Autodesk Inventor part; units mm, degrees
(part 3 of 3)
  dimension "d58" = 1
  dimension "d59" = 0.5
  dimension "d60" = 6
  dimension "d61" = 7
  dimension "d62" = 1
  dimension "d63" = 0.5
  dimension "d64" = 6
  dimension "d65" = 7
  dimension "d66" = 1
  dimension "d67" = 0.5
  dimension "d68" = 6
  dimension "d69" = 7
  dimension "d70" = 0.5
  dimension "d71" = 1
  dimension "d72" = 7
  dimension "d73" = 6
  dimension "d74" = 1
  dimension "d75" = 0.5
  dimension "d76" = 6
  dimension "d77" = 7
  dimension "d78" = 1
  dimension "d79" = 0.5
  dimension "d80" = 6
  dimension "d81" = 7
  dimension "d82" = 1
  dimension "d83" = 0.5
  constraints: 60 other
  measures "d20" distance of L2.end L0.start
  measures "d21" distance of L1.end L2.end
  measures "d22" distance between parallel lines of L4 L0
  measures "d23" distance between parallel lines of L5 L3
  measures "d24" distance of L8.end L6.start
  measures "d25" distance of L7.end L8.end
  measures "d26" distance between parallel lines of L10 L6
  measures "d27" distance between parallel lines of L11 L9
  measures "d28" distance of L14.end L12.start
  measures "d29" distance of L12.start L12.end
  measures "d30" distance between parallel lines of L16 L12
  measures "d31" distance between parallel lines of L17 L15
  measures "d32" distance of L20.end L18.start
  measures "d33" distance of L19.end L20.end
  measures "d34" distance between parallel lines of L22 L18
  measures "d35" distance between parallel lines of L23 L21
  measures "d36" distance of L25.end L26.end
  measures "d37" distance of L26.end L24.start
  measures "d38" distance between parallel lines of L28 L24
  measures "d39" distance between parallel lines of L29 L27
  measures "d40" distance of L30.start L30.end
  measures "d41" distance of L30.end L31.end
  measures "d42" distance between parallel lines of L34 L30
  measures "d43" distance between parallel lines of L35 L33
  measures "d44" distance of L37.end L38.end
  measures "d45" distance of L38.end L36.start
  measures "d46" distance between parallel lines of L40 L36
  measures "d47" distance between parallel lines of L41 L39
  measures "d48" distance of L44.end L42.start
  measures "d49" distance of L42.start L42.end
  measures "d50" distance between parallel lines of L46 L42
  measures "d51" distance between parallel lines of L47 L45
  measures "d52" distance of L50.end L48.start
  measures "d53" distance of L49.end L50.end
  measures "d54" distance between parallel lines of L52 L48
  measures "d55" distance between parallel lines of L53 L51
  measures "d56" distance of L56.end L54.start
  measures "d57" distance of L54.start L54.end
  measures "d58" distance between parallel lines of L58 L54
  measures "d59" distance between parallel lines of L59 L57
  measures "d60" distance of L62.end L60.start
  measures "d61" distance of L60.start L60.end
  measures "d62" distance between parallel lines of L64 L60
  measures "d63" distance between parallel lines of L65 L63
  measures "d64" distance of L68.end L66.start
  measures "d65" distance of L66.start L66.end
  measures "d66" distance between parallel lines of L70 L66
  measures "d67" distance between parallel lines of L71 L69
  measures "d68" distance of L74.end L72.start
  measures "d69" distance of L72.start L72.end
  measures "d70" distance between parallel lines of L76 L75
  measures "d71" distance between parallel lines of L77 L72
  measures "d72" distance of L79.end L80.end
  measures "d73" distance of L78.end L79.end
  measures "d74" distance between parallel lines of L82 L78
  measures "d75" distance between parallel lines of L83 L79
  measures "d76" distance of L84.end L85.end
  measures "d77" distance of L84.start L84.end
  measures "d78" distance between parallel lines of L88 L84
  measures "d79" distance between parallel lines of L89 L85
  measures "d80" distance of L92.end L90.start
  measures "d81" distance of L90.start L90.end
  measures "d82" distance between parallel lines of L94 L90
  measures "d83" distance between parallel lines of L95 L93
extrude "number" add sketch "Esquisse5" along normal blind 1
